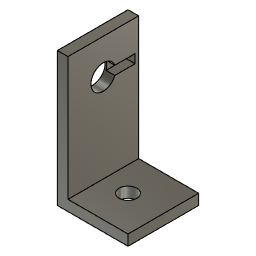
volume_pot_mount (Autodesk Fusion 360 design; units mm, degrees)
Autodesk Fusion 360 part; units mm, degrees
sketch "Sketch1" plane through (0, 0, 0) normal (0, 0, 1) x (1, 0, 0)
  line L0 (0, 0) -> (20, 0)
  line L1 (20, 0) -> (20, 20)
  line L2 (20, 20) -> (0, 20)
  line L3 (0, 20) -> (0, 0)
  line L4 (0, 0) -> (3, 0)
  line L5 (3, 0) -> (3, 20)
  line L6 (3, 20) -> (0, 20)
  line L7 (0, 20) -> (0, 0)
  line L8 (10, 0) -> (10, 20) construction
  circle A0 centre (10, 10) radius 2.5
  dimension "d7" = 20
  dimension "d8" = 20
  dimension "d9" = 3
  dimension "d10" = 20
  dimension "d12" = 5
  constraint horizontal L0
  constraint vertical L1
  constraint horizontal L2
  constraint vertical L3
  constraint coincident L0.start L3.end
  constraint horizontal L4
  constraint vertical L5
  constraint horizontal L6
  constraint vertical L7
  constraint midpoint L0 L8.start
  constraint midpoint L2 L8.end
  constraint midpoint L8 A0.centre
  measures "d7" distance of L0.start L0.end
  measures "d8" distance of L0.start L2.end
  measures "d9" distance of L0.start L4.end
  measures "d10" distance of L0.start L2.end
  measures "d12" diameter of A0
extrude "Extrude1" add sketch "Sketch1" along normal blind 3
extrude "Extrude2" add sketch "Sketch1" along normal blind 38 contours L0 L2 L3 L4 L5 L6 L7
sketch "Sketch2" plane through (0, 0, 0) normal (-1, 0, 0) x (0, -1, 0)
  line L0 (-20, 0) -> (0, 0)
  line L1 (0, 0) -> (0, 38)
  line L2 (0, 38) -> (-20, 38)
  line L3 (-20, 38) -> (-20, 0)
  line L4 (-20, 38) -> (0, 18) construction
  line L5 (-20, 38) -> (8.2843, 38) construction
  line L6 (-10, 38) -> (-10, 0) construction
  circle A0 centre (-10, 28) radius 3.5
  dimension "d17" = 45
  dimension "d18" = 7
  constraint horizontal L5
  constraint coincident L2.end L3.start
  constraint coincident L1 L4.end
  constraint midpoint L2 L6.start
  constraint midpoint L0 L6.end
  constraint midpoint L4 A0.centre
  measures "d17" angle of L4 L5
  measures "d18" diameter of A0
extrude "Extrude3" cut sketch "Sketch2" against normal up to surface (3 mm away) contours A0
sketch "Sketch3" plane through (3, 0, 0) normal (1, 0, 0) x (0, 1, 0)
  circle A0 centre (10, 28) radius 3.5
  line L0 (0, 3) -> (20, 3)
  line L1 (20, 3) -> (20, 38)
  line L2 (20, 38) -> (0, 38)
  line L3 (0, 38) -> (0, 3)
  line L4 (10, 28) -> (10, 29.25)
  line L5 (10, 29.25) -> (19, 29.25)
  line L6 (19, 29.25) -> (19, 26.75)
  line L7 (19, 26.75) -> (10, 26.75)
  line L8 (10, 26.75) -> (10, 29.25)
  dimension "d21" = 1.25
  dimension "d23" = 9
  dimension "d24" = 2.5
  constraint coincident A0.centre L4.start
  constraint perpendicular L2 L4
  constraint horizontal L5
  constraint vertical L6
  constraint horizontal L7
  constraint vertical L8
  measures "d21" distance of A0.centre L4.end
  measures "d23" distance of L4.end L5.end
  measures "d24" distance of L4.end L7.end
extrude "Extrude4" cut sketch "Sketch3" against normal blind 2.5 contours A0 L5 L6 L7
equation "pot_hole_diameter = 7 mm"
equation "pot_turn_stop_slot_depth = 2.5 mm"
equation "pot_turn_stop_slot_width = 2.5 mm"
equation "thickness = 3 mm"
equation "mount_width = 20 mm"
equation "mount_height = 35 mm"
equation "d7 = mount_width"
equation "d8 = mount_width"
equation "d9 = thickness"
equation "d10 = mount_width"
equation "screw_hole_diameter = 5 mm"
equation "d12 = screw_hole_diameter"
equation "d13 = thickness"
equation "d15 = thickness + mount_height"
equation "d18 = pot_hole_diameter"
equation "d21 = pot_turn_stop_slot_width / 2"
equation "pot_slot_length = 9 mm"
equation "d23 = pot_slot_length"
equation "d24 = pot_turn_stop_slot_width"
equation "d25 = -pot_turn_stop_slot_depth"
